Autodesk Inventor part; units mm, degrees
(part 2 of 2)
sketch "Sketch35" plane through (0, 0, 8) normal (0, 0, 1) x (1, 0, 0)
  circle A0 centre (-52.625, 102) radius 2 projected
  circle A1 centre (-52.625, 90) radius 2 projected
  circle A2 centre (-34.125, 90) radius 2 projected
  circle A3 centre (-34.125, 102) radius 2 projected
  circle A4 centre (28.625, 121) radius 2 projected
  circle A5 centre (16.625, 121) radius 2 projected
  circle A6 centre (16.625, 137) radius 2 projected
  circle A7 centre (42.875, 125) radius 1.5 projected
  circle A8 centre (58.625, 121) radius 2 projected
  circle A9 centre (-43.75, 62) radius 2 projected
  circle A10 centre (-43.75, 22) radius 2 projected
  circle A11 centre (-43.75, -18) radius 2 projected
  circle A12 centre (-43.75, -58) radius 2 projected
  circle A13 centre (52.125, -58) radius 1.5 projected
  circle A14 centre (52.125, -38) radius 1.5 projected
  circle A15 centre (52.125, -18) radius 1.5 projected
  circle A16 centre (52.125, 2) radius 1.5 projected
  circle A17 centre (52.125, 22) radius 1.5 projected
  circle A18 centre (52.125, 42) radius 1.5 projected
  circle A19 centre (52.125, 62) radius 1.5 projected
  circle A20 centre (52.125, 82) radius 1.5 projected
  circle A21 centre (52.125, 102) radius 1.5 projected
  circle A22 centre (16.625, -61) radius 1.5 projected
  line L0 (-32.125, 155) -> (-32.125, 112.5) projected
  line L1 (-32.125, 112.5) -> (-39.625, 112.5) projected
  line L2 (-39.625, 110) -> (-39.625, 112.5) projected
  line L3 (-39.625, 110) -> (-56.625, 110) projected
  line L4 (-56.625, 110) -> (-56.625, 87.5) projected
  line L5 (-56.625, 87.5) -> (-55.375, 87.5) projected
  line L6 (-55.375, 87.5) -> (-55.375, 82) projected
  line L7 (-55.375, 82) -> (-47.875, 82) projected
  line L8 (-47.875, 82) -> (-47.875, -65) projected
  line L9 (-47.875, -65) -> (56.625, -65) projected
  line L10 (56.625, -65) -> (56.625, 105) projected
  line L11 (64.625, 113) -> (56.625, 105) projected
  line L12 (64.625, 113) -> (64.625, 129) projected
  line L13 (64.625, 129) -> (21.625, 129) projected
  line L14 (21.625, 129) -> (21.625, 150) projected
  line L15 (18.3571, 150) -> (21.625, 150) projected
  arc A23 (14.8929, 150) -> (18.3571, 150) centre (16.625, 149) ccw projected
  line L16 (13.375, 150) -> (14.8929, 150) projected
  line L17 (13.375, 150) -> (13.375, 116.5) projected
  line L18 (9.375, 112.5) -> (13.375, 116.5) projected
  line L19 (9.375, 112.5) -> (2.375, 112.5) projected
  line L20 (0.375, 110.5) -> (2.375, 112.5) projected
  line L21 (0.375, 110.5) -> (0.375, 85) projected
  line L22 (-16.625, 85) -> (0.375, 85) projected
  line L23 (-16.625, 85) -> (-16.625, 110.5) projected
  line L24 (-18.625, 112.5) -> (-16.625, 110.5) projected
  line L25 (-18.625, 112.5) -> (-25.625, 112.5) projected
  line L26 (-29.625, 116.5) -> (-25.625, 112.5) projected
  line L27 (-29.625, 116.5) -> (-29.625, 155) projected
  line L28 (-32.125, 155) -> (-29.625, 155) projected
  circle A24 centre (-3.25, -55) radius 3.75 projected
  circle A25 centre (26.5, -55) radius 3.75 projected
  circle A26 centre (-33, -55) radius 3.75 projected
  line L29 (-13.875, 65.6) -> (-13.875, 60.1495) projected
  arc A27 (-0.375, 79.1) -> (-13.875, 65.6) centre (-0.375, 65.6) ccw projected
  line L30 (8.9856, 79.1) -> (-0.375, 79.1) projected
  arc A28 (8.9856, 79.1) -> (9.2663, 79.1862) centre (8.9856, 79.6) ccw projected
  arc A29 (24.9837, 79.1862) -> (9.2663, 79.1862) centre (17.125, 67.6) ccw projected
  arc A30 (24.9837, 79.1862) -> (25.2644, 79.1) centre (25.2644, 79.6) ccw projected
  line L31 (34.625, 79.1) -> (25.2644, 79.1) projected
  arc A31 (48.125, 65.6) -> (34.625, 79.1) centre (34.625, 65.6) ccw projected
  line L32 (48.125, 60.1495) -> (48.125, 65.6) projected
  line L33 (42.7709, 48.7505) -> (48.125, 60.1495) projected
  arc A32 (42.7709, 48.7505) -> (42.7235, 48.5379) centre (43.2235, 48.5379) ccw projected
  line L34 (42.7235, 42.9489) -> (42.7235, 48.5379) projected
  arc A33 (40.9627, 36.2825) -> (42.7235, 42.9489) centre (29.2235, 42.9489) ccw projected
  line L35 (36.7894, 28.9336) -> (40.9627, 36.2825) projected
  arc A34 (25.0502, 22.1) -> (36.7894, 28.9336) centre (25.0502, 35.6) ccw projected
  line L36 (9.1998, 22.1) -> (25.0502, 22.1) projected
  arc A35 (-2.5394, 28.9336) -> (9.1998, 22.1) centre (9.1998, 35.6) ccw projected
  line L37 (-6.7127, 36.2825) -> (-2.5394, 28.9336) projected
  arc A36 (-8.4735, 42.9489) -> (-6.7127, 36.2825) centre (5.0265, 42.9489) ccw projected
  line L38 (-8.4735, 48.5379) -> (-8.4735, 42.9489) projected
  arc A37 (-8.4735, 48.5379) -> (-8.5209, 48.7505) centre (-8.9735, 48.5379) ccw projected
  line L39 (-13.875, 60.1495) -> (-8.5209, 48.7505) projected
  line L40 (-38.875, -38) -> (34.375, -38)
  line L41 (34.375, -38) -> (34.375, 17.1)
  line L42 (34.375, 17.1) -> (-38.875, 17.1)
  line L43 (-38.875, 17.1) -> (-38.875, -38)
  line L44 (-38.875, -38) -> (34.375, 17.1)
  line L45 (34.375, -38) -> (-38.875, 17.1)
  line L46 (41.375, 107) -> (41.375, -45) projected
  line L47 (41.2938, -39.4504) -> (-45.7268, 26.008)
  line L48 (37.2958, -43.951) -> (-40.874, 14.8497)
  line L49 (-45.7938, -39.4504) -> (32.376, 19.3503)
  line L50 (-41.7958, -43.951) -> (36.374, 14.8497)
  line L51 (41.375, -45) -> (-29.625, -45) projected
  line L52 (-13.4735, 47.5337) -> (-13.4735, 42.9489)
  arc A38 (-13.4735, 42.9489) -> (-11.0605, 33.8134) centre (5.0265, 42.9489) ccw
  line L53 (-11.0605, 33.8134) -> (-6.8872, 26.4645)
  arc A39 (-6.8872, 26.4645) -> (9.1998, 17.1) centre (9.1998, 35.6) ccw
  line L54 (9.1998, 17.1) -> (25.0502, 17.1)
  arc A40 (25.0502, 17.1) -> (41.1372, 26.4645) centre (25.0502, 35.6) ccw
  line L55 (41.1372, 26.4645) -> (45.3105, 33.8134)
  arc A41 (45.3105, 33.8134) -> (47.7235, 42.9489) centre (29.2235, 42.9489) ccw
  line L56 (47.7235, 42.9489) -> (47.7235, 47.5337)
  line L57 (47.7235, 47.5337) -> (53.125, 59.0337)
  line L58 (53.125, 59.0337) -> (53.125, 65.6)
  arc A42 (53.125, 65.6) -> (34.625, 84.1) centre (34.625, 65.6) ccw
  line L59 (34.625, 84.1) -> (26.5457, 84.1)
  arc A43 (26.5457, 84.1) -> (7.7043, 84.1) centre (17.125, 67.6) ccw
  line L60 (7.7043, 84.1) -> (-0.375, 84.1)
  arc A44 (-0.375, 84.1) -> (-18.875, 65.6) centre (-0.375, 65.6) ccw
  line L61 (-18.875, 65.6) -> (-18.875, 59.0337)
  line L62 (-18.875, 59.0337) -> (-13.4735, 47.5337)
  line L63 (-38.875, 17.1) -> (-38.875, 78)
  line L64 (-38.875, 78) -> (-14.1042, 78)
  line L65 (34.375, 20.1) -> (-38.875, 20.1)
  line L66 (34.375, 14.1) -> (-38.875, 14.1)
  line L67 (-38.875, 20.1) -> (-17.5092, 72.5762)
  line L68 (-38.875, 78) -> (-1.0941, 17.1)
  line L69 (-36.3257, 79.5815) -> (1.4552, 18.6815)
  line L70 (-41.4243, 76.4185) -> (-3.6434, 15.5185)
  line L71 (-14.7307, 71.4451) -> (-41.5539, 5.5648)
  line L72 (-20.2878, 73.7075) -> (-43.5761, 16.5093)
  point P0 (0, 0)
  point P1 (-2.25, -10.45)
  point P2 (17.125, 22.1)
  point P3 (-2.25, -38)
  point P4 (34.375, 13.346)
  point P5 (2.7406, -10.45)
  point P6 (34.375, -34.246)
  point P7 (-2.25, -6.696)
  point P8 (29.3844, 17.1)
  point P9 (-33.8844, 17.1)
  point P10 (-38.875, -34.246)
  point P11 (-7.2406, -10.45)
  point P12 (-38.875, 13.346)
  point P13 (-2.25, -14.204)
  point P14 (-33.8844, -38)
  point P15 (29.3844, -38)
  point P16 (-18.875, 61.2662)
  point P17 (-21.2875, 55.341)
  point P18 (-13.4723, 42.7436)
  point P19 (-35.3446, 78)
  point P20 (-23.2431, 58.4933)
  point P21 (-38.875, 28.0556)
  point P22 (-27.9966, 54.774)
  point P23 (-38.875, 72.3092)
  point P24 (-24.0853, 48.4693)
  point P25 (-35.6359, 20.1)
  point P26 (-6.4856, 20.1)
  point P27 (25.3962, 14.1)
  point P28 (-29.8962, 14.1)
  dimension "d245" = 5
  dimension "d247" = 9
  dimension "d249" = 7
  dimension "d250" = 3
  dimension "d251" = 3
  dimension "d252" = 3
  dimension "d253" = 3
  dimension "d254" = 7
  dimension "d258" = 7
  dimension "d259" = 3
  dimension "d260" = 3
  dimension "d261" = 3
  dimension "d262" = 3
  dimension "d263" = 3
  dimension "d264" = 3
  constraints: 62 end point, 16 point on circle, 11 parallel, 7 centre point, 4 midpoint, 3 point on line, 2 horizontal, 2 tangent, 1 collinear, 1 perpendicular, 17 other
  measures "d245" distance from line of L42 point (17.125, 22.1)
  measures "d247" distance between parallel lines of L8 L43
  measures "d249" distance between parallel lines of L46 L41
  measures "d250" distance between parallel lines of L45 L47
  measures "d251" distance between parallel lines of L48 L45
  measures "d252" distance between parallel lines of L44 L50
  measures "d253" distance between parallel lines of L44 L49
  measures "d254" distance between parallel lines of L51 L40
  measures "d258" distance from line of L22 L63.end
  measures "d259" distance between parallel lines of L65 L42
  measures "d260" distance between parallel lines of L66 L42
  measures "d261" distance between parallel lines of L71 L67
  measures "d262" distance between parallel lines of L67 L72
  measures "d263" distance between parallel lines of L70 L68
  measures "d264" distance between parallel lines of L68 L69
extrude "Extrusion25" cut sketch "Sketch35" against normal through all contours A44 L67 L69 L64 | L49 L47 L66 | L70 L72 L63 | L41 L47 L50 | L49 L43 L71 L48 | L65 L71 L70 | L71 L43 L48 | L40 L50 L48
fillet "Fillet4" radius 3 21 edges at (-33.8844, -38, 2.5) (-38.875, -34.246, 2.5) (-38.875, 13.346, 2.5) (-2.25, -6.696, 2.5) (-7.2406, -10.45, 2.5) (-2.25, -14.204, 2.5) (2.7406, -10.45, 2.5) (29.3844, -38, 2.5) (34.375, -34.246, 2.5) (34.375, 13.346, 2.5) (-29.8962, 14.1, 2.5) (25.3962, 14.1, 2.5) (-35.6359, 20.1, 2.5) (-24.0853, 48.4693, 2.5) (-38.875, 28.0556, 2.5) (-6.4856, 20.1, 2.5) (-38.875, 72.3092, 2.5) (-27.9966, 54.774, 2.5) (-35.3446, 78, 2.5) (-14.1042, 78, 2.5) (-23.2431, 58.4933, 2.5)
equation "\"d114\" = 0.5 * d112"
equation "\"d124\" = d120"
equation "\"d130\" = d129"
equation "\"d131\" = d130"
equation "\"d143\" = 0.5 * d142"
equation "\"d178\" = d177"
equation "\"d168\" = 2 * d167"
equation "\"d169\" = d168"
equation "\"d167\" = 0.166667 * d166"
equation "\"d166\" = 89.25"
body "Solid1"
